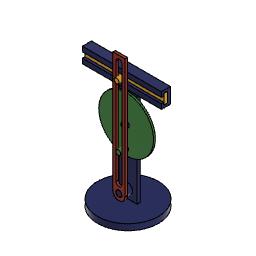
Crank and Slotted Link v5 (Autodesk Fusion 360 design; units mm, degrees)
Autodesk Fusion 360 part; units mm, degrees
sketch "holder stand" plane through (0, 0, 0) normal (0, 0, 1) x (1, 0, 0)
  circle A0 centre (0, 0) radius 50
  dimension "d1" = 100
  constraint coincident A0.centre origin
  measures "d1" diameter of A0
extrude "Extrude1" add sketch "holder stand" along normal blind 10 makes body 1
sketch "holder" plane through (0, 0, 10) normal (0, 0, 1) x (-1, 0, 0)
  circle A0 centre (0, 0) radius 50
  line L0 (0, 0) -> (-15, 0)
  line L1 (-15, 0) -> (-15, -5)
  line L2 (-15, -5) -> (0, -5)
  line L3 (0, -5) -> (0, 0)
  line L4 (0, 0) -> (15, 0)
  line L5 (15, -5) -> (0, -5)
  line L6 (15, 0) -> (15, -5)
  dimension "d4" = 15
  dimension "d5" = 5
  constraint horizontal L0
  constraint vertical L1
  constraint horizontal L2
  constraint vertical L3
  constraint coincident A0.centre L0.start
  constraint symmetric A0.centre L3 L0.start
  constraint symmetric L0.end L3 L4.end
  constraint symmetric L1.end L3 L5.start
  constraint symmetric L2.end L3 L5.end
  measures "d4" distance of A0.centre L0.end
  measures "d5" distance of A0.centre L2.end
extrude "Extrude2" cut sketch "holder" against normal blind 10 contours L0 L1 L2 L3 | L3 L4 L5 L6 bodies 1
extrude "Extrude3" add sketch "holder" along normal blind 190 separate body contours L0 L1 L2 L3 | L3 L4 L5 L6 makes body 2
extrude "Extrude4" add 1 faces at (5, 3.3333, 10) along direction (0, 0, -1) blind 10 on bodies 2 bodies 2
sketch "crank holder" plane through (0, 0, 0) normal (0, -1, 0) x (1, 0, 0)
  line L0 (15, 0) -> (15, 200)
  line L1 (15, 200) -> (-15, 200)
  line L2 (-15, 200) -> (-15, 0)
  line L3 (-15, 0) -> (15, 0)
  line L4 (0, 200) -> (0, 118) construction
  circle A0 centre (0, 118) radius 5
  dimension "d12" = 82
  dimension "d13" = 10
  constraint midpoint L1 L4.start
  constraint perpendicular L1 L4
  constraint coincident L4.end A0.centre
  measures "d12" distance of L4.start L4.end
  measures "d13" diameter of A0
extrude "Extrude5" add sketch "crank holder" along normal blind 7 contours A0 bodies 2
sketch "crank" plane through (0, -7, 0) normal (0, -1, 0) x (1, 0, 0)
  circle A0 centre (0, 118) radius 5
  circle A1 centre (0, 118) radius 45
  dimension "d16" = 90
  constraint concentric A0 A1
  measures "d16" diameter of A1
extrude "Extrude6" add sketch "crank" along normal blind 3 separate body makes body 3
move_body "Move1" bodies 3 to x (1, 0, 0) y (0, 1, 0) z (0, 0, 1) at (0, 7, 0)
move_face "OffsetFaces1" offset -0.3 1 faces at (4.9752, -4.6667, 117.5022) on bodies 2
sketch "slider holder right" plane through (15, 0, 0) normal (1, 0, 0) x (0, 1, 0)
  line L0 (5, 0) -> (5, 200)
  line L1 (5, 200) -> (0, 200)
  line L2 (0, 200) -> (0, 0)
  line L3 (0, 0) -> (5, 0)
  line L4 (0, 200) -> (5, 200)
  line L5 (5, 200) -> (5, 175)
  line L6 (5, 175) -> (0, 175)
  line L7 (0, 175) -> (0, 200)
  dimension "d20" = 25
  constraint horizontal L4
  constraint vertical L5
  constraint horizontal L6
  constraint vertical L7
  constraint coincident L1.end L2.start
  measures "d20" distance of L1.end L6.end
sketch "slider holder left" plane through (-15, 0, 0) normal (-1, 0, 0) x (0, -1, 0)
  line L0 (0, 0) -> (0, 200)
  line L1 (0, 200) -> (-5, 200)
  line L2 (-5, 200) -> (-5, 0)
  line L3 (-5, 0) -> (0, 0)
  line L4 (-5, 200) -> (0, 200)
  line L5 (0, 200) -> (0, 175)
  line L6 (0, 175) -> (-5, 175)
  line L7 (-5, 175) -> (-5, 200)
  constraint horizontal L4
  constraint vertical L5
  constraint horizontal L6
  constraint vertical L7
  constraint coincident L0 L5.end
  constraint coincident L1.end L2.start
extrude "Extrude7" add sketch "slider holder right" along normal blind 50 contours L0 L1 L2 L4 L5 L6 L7 bodies 2
extrude "Extrude8" add sketch "slider holder left" along normal blind 50 contours L0 L1 L2 L4 L5 L6 L7 bodies 2
sketch "slider holder front" plane through (0, 0, 0) normal (0, -1, 0) x (1, 0, 0)
  circle A0 centre (0, 118) radius 4.7
  line L0 (15, 0) -> (15, 175)
  line L1 (15, 175) -> (65, 175)
  line L2 (65, 175) -> (65, 200)
  line L3 (65, 200) -> (-65, 200)
  line L4 (-65, 200) -> (-65, 175)
  line L5 (-65, 175) -> (-15, 175)
  line L6 (-15, 175) -> (-15, 0)
  line L7 (-15, 0) -> (15, 0)
  line L8 (-65, 200) -> (65, 200)
  line L9 (65, 200) -> (65, 196)
  line L10 (65, 196) -> (-65, 196)
  line L11 (-65, 196) -> (-65, 200)
  line L12 (-65, 175) -> (65, 175)
  line L13 (65, 175) -> (65, 179)
  line L14 (65, 179) -> (-65, 179)
  line L15 (-65, 179) -> (-65, 175)
  dimension "d25" = 4
  dimension "d26" = 4
  constraint horizontal L8
  constraint vertical L9
  constraint horizontal L10
  constraint vertical L11
  constraint coincident L3.end L4.start
  constraint horizontal L12
  constraint vertical L13
  constraint horizontal L14
  constraint vertical L15
  constraint coincident L4.end L5.start
  measures "d25" distance of L3.end L10.end
  measures "d26" distance of L4.end L14.end
extrude "Extrude9" add sketch "slider holder front" along normal blind 10 contours L1 L2 L4 L5 L12 L13 L14 L15 | L2 L3 L4 L8 L9 L10 L11 bodies 2
sketch "slider holder bottom" plane through (0, 0, 179) normal (0, 0, 1) x (-1, 0, 0)
  line L0 (-65, 0) -> (65, 0)
  line L1 (65, 0) -> (65, 10)
  line L2 (65, 10) -> (-65, 10)
  line L3 (-65, 10) -> (-65, 0)
  line L4 (65, 10) -> (-65, 10)
  line L5 (-65, 10) -> (-65, 6)
  line L6 (-65, 6) -> (65, 6)
  line L7 (65, 6) -> (65, 10)
  dimension "d29" = 4
  constraint horizontal L4
  constraint vertical L5
  constraint horizontal L6
  constraint vertical L7
  constraint coincident L1.end L2.start
  measures "d29" distance of L1.end L6.end
sketch "slider holder top" plane through (0, 0, 196) normal (0, 0, -1) x (1, 0, 0)
  line L0 (-65, 0) -> (65, 0)
  line L1 (65, 0) -> (65, 10)
  line L2 (65, 10) -> (-65, 10)
  line L3 (-65, 10) -> (-65, 0)
  line L4 (-65, 10) -> (65, 10)
  line L5 (65, 10) -> (65, 6)
  line L6 (65, 6) -> (-65, 6)
  line L7 (-65, 6) -> (-65, 10)
  dimension "d30" = 4
  constraint horizontal L4
  constraint vertical L5
  constraint horizontal L6
  constraint vertical L7
  constraint coincident L2.end L3.start
  measures "d30" distance of L2.end L6.end
extrude "Extrude10" add sketch "slider holder top" along normal blind 4 contours L1 L2 L3 L4 L5 L6 L7 bodies 2
extrude "Extrude11" add sketch "slider holder bottom" along normal blind 4 contours L1 L2 L3 L4 L5 L6 L7 bodies 2
sketch "slider" plane through (0, 0, 0) normal (1, 0, 0) x (0, 1, 0)
  line L0 (-6, 196) -> (0, 196)
  line L1 (0, 196) -> (0, 179)
  line L2 (0, 179) -> (-6, 179)
  line L3 (-6, 179) -> (-6, 196)
  constraint horizontal L0
  constraint vertical L1
  constraint horizontal L2
  constraint vertical L3
extrude "Extrude12" add sketch "slider" against normal blind 130 separate body makes body 4
move_body "Move2" bodies 4 to x (1, 0, 0) y (0, 1, 0) z (0, 0, 1) at (65, 0, 0)
move_face "OffsetFaces2" offset -0.2 4 faces at (21.6667, -6, 184.6667) (21.6667, -4, 196) (21.6667, 0, 190.3333) (21.6667, -2, 179) on bodies 4
sketch "link holder" plane through (0, 0, 0) normal (0, -1, 0) x (1, 0, 0)
  line L0 (15, 175) -> (-15, 175)
  line L1 (-15, 175) -> (-15, 0)
  line L2 (-15, 0) -> (15, 0)
  line L3 (15, 0) -> (15, 175)
  circle A0 centre (0, 118) radius 4.7
  circle A1 centre (0, 25) radius 5
  dimension "d38" = 10
  measures "d38" diameter of A1
extrude "Extrude13" add sketch "link holder" along normal blind 15 contours A1 bodies 2
sketch "slotted link" plane through (0, -15, 0) normal (0, -1, 0) x (1, 0, 0)
  circle A0 centre (0, 25) radius 5
  circle A1 centre (0, 25) radius 10
  line L0 (-9.9664, 24.181) -> (10, 24.181)
  line L1 (10, 24.181) -> (10, 222)
  line L2 (10, 222) -> (-9.9664, 222)
  line L3 (-9.9664, 222) -> (-9.9664, 24.181)
  line L4 (-4.9325, 24.181) -> (5, 24.181)
  circle A2 centre (0.0338, 40) radius 4.9662
  line L5 (-4.9325, 24.181) -> (5, 24.181)
  line L6 (5, 24.181) -> (5, 217.0303)
  line L7 (5, 217.0303) -> (-4.9325, 217.0303)
  line L8 (-4.9325, 217.0303) -> (-4.9325, 24.181)
  circle A3 centre (0, 212.0303) radius 5
  dimension "d41" = 5
  constraint horizontal L0
  constraint vertical L1
  constraint horizontal L2
  constraint vertical L3
  constraint coincident A1 L0.start
  constraint horizontal L4
  constraint coincident L0 L4.start
  constraint coincident A0 L4.start
  constraint horizontal L5
  constraint vertical L6
  constraint horizontal L7
  constraint vertical L8
  constraint tangent L7 A3
  constraint tangent L6 A3
  constraint tangent A0 L6
  constraint tangent A2 L6
  constraint tangent A2 L8
  measures "d41" distance of A0
extrude "Extrude14" add sketch "slotted link" against normal blind 4 separate body contours A1 L0 L6 | A0 A1 L6 L8 | A0 A1 L0 L3 L8 | A0 A1 L0 L4 L5 | A1 L1 L2 L3 L6 L7 L8 A3 | A1 A2 L6 L8 | L6 L7 A3 | L7 L8 A3 makes body 5
move_face "OffsetFaces3" offset -0.3 1 faces at (4.9752, -10, 24.5022) on bodies 2
sketch "slotted link holder" plane through (0, -15, 0) normal (0, -1, 0) x (1, 0, 0)
  circle A0 centre (0, 25) radius 4.7
  circle A1 centre (0, 25) radius 7.5
  dimension "d46" = 15
  constraint concentric A0 A1
  measures "d46" diameter of A1
extrude "Extrude15" add sketch "slotted link holder" along normal blind -15 and the other way blind 4 bodies 2
sketch "crank pin" plane through (0, -3, 0) normal (0, -1, 0) x (1, 0, 0)
  circle A0 centre (0, 118) radius 5
  circle A1 centre (0, 118) radius 45
  circle A2 centre (0, 84) radius 4
  dimension "d51" = 8
  measures "d51" diameter of A2
sketch "slider pin" plane through (0, -5.8, 0) normal (0, -1, 0) x (1, 0, 0)
  line L0 (65, 179.2) -> (65, 195.8)
  line L1 (65, 195.8) -> (-65, 195.8)
  line L2 (-65, 195.8) -> (-65, 179.2)
  line L3 (-65, 179.2) -> (65, 179.2)
  circle A0 centre (0, 187.5) radius 4
  dimension "d52" = 8
  measures "d52" diameter of A0
extrude "Extrude16" add sketch "slider pin" along normal blind 13 contours A0 bodies 4
extrude "Extrude17" add sketch "crank pin" along normal blind 13 contours A2 bodies 3
copy_body "Body->Comp1" bodies 1 removing the originals makes body 6 in component "holder stand"
copy_body "Body->Comp2" bodies 2 removing the originals makes body 7 in component "holder"
copy_body "Body->Comp3" bodies 3 removing the originals makes body 8 in component "crank"
copy_body "Body->Comp4" bodies 4 removing the originals makes body 9 in component "slider"
copy_body "Body->Comp5" bodies 5 removing the originals makes body 10 in component "slotted link"
component "holder stand" placed x (1, 0, 0) y (0, 1, 0) z (0, 0, 1) at (0, 0, 0)
component "holder" placed x (1, 0, 0) y (0, 1, 0) z (0, 0, 1) at (0, 0, 0)
component "crank" placed x (1, 0, 0) y (0, 1, 0) z (0, 0, 1) at (0, 0, 0)
component "slider" placed x (1, 0, 0) y (0, 1, 0) z (0, 0, 1) at (0, 0, 0)
component "slotted link" placed x (1, 0, 0) y (0, 1, 0) z (0, 0, 1) at (0, 0, 0)
named bodies: "holder stand", "holder", "crank", "slider", "slotted link"
